small_spool_v3 (Autodesk Fusion 360 design; units mm, degrees)
Autodesk Fusion 360 part; units mm, degrees
sketch "Esquisse1" plane through (0, 0, 0) normal (0, 0, 1) x (1, 0, 0)
  circle A0 centre (0, 0) radius 1.75
  circle A1 centre (0, 0) radius 4
  circle A2 centre (0, 0) radius 7
  dimension "d1" = 3.5
  dimension "d10" = 8
  dimension "d11" = 3
  constraint coincident A0.centre A1.centre
  measures "d1" diameter of A0
  measures "d10" diameter of A1
extrude "Extrusion2" add sketch "Esquisse1" along normal blind 5 contours A1
extrude "Extrusion3" add sketch "Esquisse1" along normal blind 2 contours A2
mirror "Symétrie miroir2" about plane through (0, 0, 5) normal (0, 0, 1) of bodies 1 merged
